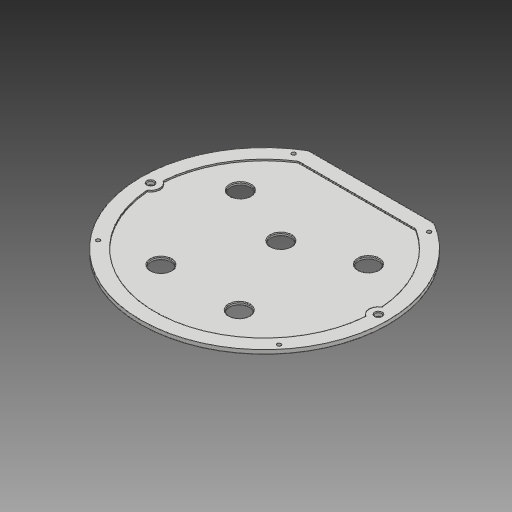
# Autodesk Inventor part: Gehäuse Unterplatte
Saved by Autodesk Inventor 2019.4 (Build 234330000, 330)
## iProperties
Part Number: Gehäuse Unterplatte
Material: Generisch
Document SubType Name: Modeling
Designer: rYan
Density: 1 g/cm^3
Appearance: Vorgabe
Mass: 48.9318 g
Surface Area: 477.374 cm^2
Volume: 48.9318 cm^3
Author: rYan
Autodesk Inventor part; units mm, degrees
ref_plane "YZ Plane" through (0, 0, 0) normal (1, 0, 0) x (0, 1, 0)
ref_plane "XZ Plane" through (0, 0, 0) normal (0, 1, 0) x (-1, 0, 0)
ref_plane "XY Plane" through (0, 0, 0) normal (0, 0, 1) x (1, 0, 0)
sketch "Skizze1" plane through (0, 0, 0) normal (0, 0, 1) x (1, 0, 0)
  arc A0 (-44.0908, 75) -> (44.0908, 75) centre (0, 0) ccw
  line L0 (-44.0908, 75) -> (44.0908, 75)
  dimension "d0" = 174
  dimension "d1" = 75
  constraints: 2 end point, 2 point on circle, 1 centre point, 1 coincident, 1 horizontal
  measures "d0" diameter of A0
  measures "d1" distance from line of point (0, 0) L0
extrude "Extrusion1" add sketch "Skizze1" along normal blind 2
sketch "Skizze2" plane through (0, 0, 2) normal (0, 0, 1) x (1, 0, 0)
  arc A0 (-44.0908, 75) -> (44.0908, 75) centre (0, 0) ccw projected
  line L0 (44.0908, 75) -> (-44.0908, 75) projected
  arc A1 (-41.2795, 65) -> (41.2795, 65) centre (0, 0) ccw
  line L1 (-41.2795, 65) -> (41.2795, 65)
  dimension "d4" = 10
  constraints: 2 end point, 2 point on circle, 1 centre point, 1 other
  measures "d4" radial gap between concentric circles of A0 A1
extrude "Extrusion2" add sketch "Skizze2" along normal blind 1
sketch "Skizze8" plane through (0, 0, 2) normal (0, 0, 1) x (1, 0, 0)
  line L0 (41.2795, 65) -> (-41.2795, 65) projected
  arc A0 (-41.2795, 65) -> (41.2795, 65) centre (0, 0) ccw projected
  circle A1 centre (0, 0) radius 80 construction
  circle A2 centre (-80, 0) radius 6.5
  circle A3 centre (80, 0) radius 6.5
  line L1 (-121.8, 0) -> (121.8, 0) projected
  dimension "d38" = 160
  dimension "d39" = 13
  dimension "d40" = 13
  constraints: 3 centre point, 2 point on circle, 2 point on line, 1 coincident
  measures "d38" diameter of A1
  measures "d39" diameter of A2
  measures "d40" diameter of A3
extrude "Extrusion4" add sketch "Skizze8" along normal blind 1 contours A3 L1 A0 | A0 L1 A3 | A2 L1 A0 | A0 L1 A2 | L1 A3 A0 | A0 A3 L1 | L1 A2 A0 | A0 A2 L1
sketch "Skizze3" plane through (0, 0, 3) normal (0, 0, 1) x (1, 0, 0)
  line L0 (0, 107.4) -> (0, -119.4) projected
  line L1 (-121.8, 0) -> (121.8, 0) projected
  point P0 (0, 0)
  point P1 (-80, 0)
  point P2 (80, 0)
  dimension "d7" = 160
  constraints: 2 point on line, 1 symmetric about line
  measures "d7" distance of point (80, 0) point (-80, 0)
hole "Bohrung1" at (-80, 0, 3) at (80, 0, 3) direction (0, 0, -1) diameter 4.4 end through all
sketch "Skizze4" plane through (0, 0, 3) normal (0, 0, 1) x (1, 0, 0)
  circle A0 centre (0, 0) radius 83 construction
  line L0 (0, 0) -> (-47.6068, 67.9896) construction
  line L1 (0, 0) -> (-63.5817, -53.3514) construction
  line L2 (0, 117) -> (0, -121) projected
  line L3 (-121.8, 0) -> (121.8, 0) projected
  point P0 (63.5817, -53.3514)
  point P1 (47.6068, 67.9896)
  dimension "d15" = 166
  dimension "d16" = 55
  dimension "d17" = 40
  constraints: 4 end point, 4 point on circle, 2 coincident, 2 symmetric about line, 1 centre point
  measures "d15" diameter of A0
  measures "d16" angle of L0 L3
  measures "d17" angle of L3 L1
hole "Bohrung2" at (-63.5817, -53.3514, 3) at (-47.6068, 67.9896, 3) at (63.5817, -53.3514, 3) at (47.6068, 67.9896, 3) direction (0, 0, -1) diameter 2.75 end through all
sketch "Skizze5" plane through (0, 0, 0) normal (0, 0, -1) x (-1, 0, 0)
  line L0 (0, -119.4) -> (0, 107.4) projected
  line L1 (-121.8, 0) -> (121.8, 0) projected
  point P0 (0, 0)
  point P1 (-45, 28)
  point P2 (-27.5, -45.25)
  point P3 (45, 28)
  point P4 (27.5, -45.25)
  point P5 (0, 11.5)
  dimension "d113" = 45
  dimension "d114" = 28
  dimension "d115" = 27.5
  dimension "d116" = 45.25
  dimension "d117" = 11.5
  constraints: 2 symmetric about line, 1 point on line
  measures "d113" distance from line of L0 point (-45, 28)
  measures "d114" distance from line of L1 point (-45, 28)
  measures "d115" distance from line of point (-27.5, -45.25) L0
  measures "d116" distance from line of point (-27.5, -45.25) L1
  measures "d117" distance from line of L1 point (0, 11.5)
hole "Bohrung3" at (45, 28, 0) at (27.5, -45.25, 0) at (0, 11.5, 0) at (-45, 28, 0) at (-27.5, -45.25, 0) direction (0, 0, 1) diameter 14 end through all
fillet "Rundung1" radius 2 4 edges at (-44.0908, 75, 1.5) (44.0908, 75, 1.5) (41.2795, 65, 2.5) (-41.2795, 65, 2.5)
sketch "Skizze17" plane through (0, 0, 0) normal (0, 0, -1) x (-1, 0, 0)
  line L0 (-43.5431, 75) -> (43.5431, 75) projected
  line L1 (28.5, 75) -> (-28.5, 75)
  line L2 (-28.5, 75) -> (-28.5, -28.5)
  line L3 (-28.5, -28.5) -> (28.5, -28.5)
  line L4 (28.5, -28.5) -> (28.5, 75)
  line L5 (0, -119.4) -> (0, 107.4) projected
  line L6 (-43.5431, 75) -> (43.5431, 75) projected
  line L7 (-30.5, 75) -> (30.5, 75)
  line L8 (30.5, 75) -> (30.5, -30.5)
  line L9 (30.5, -30.5) -> (-30.5, -30.5)
  line L10 (-30.5, -30.5) -> (-30.5, 75)
  point P0 (0, 0)
  point P1 (-5, 75)
  dimension "d107" = 28.5
  dimension "d108" = 57
  dimension "d109" = 2
  dimension "d110" = 2
  constraints: 16 end point, 4 parallel, 2 horizontal, 2 perpendicular, 2 point on line, 2 other
  measures "d107" distance from line of L3 point (0, 0)
  measures "d108" distance of L2.end L3.end
  measures "d109" distance between parallel lines of L10 L2
  measures "d110" distance between parallel lines of L3 L9
extrude "Extrusion10" cut sketch "Skizze17" against normal blind 1 contours L0 L2 L3 L5 L9 L10 | L5 L3 L4 L0 L8 L9
chamfer "Fase1" distance 0.3 angle 45 17 edges at (-27.5, -52.25, 0) (27.5, -52.25, 0) (-45, 21, 0) (45, 21, 0) (0, 4.5, 0) (-63.5817, -51.9764, 0) (63.5817, -51.9764, 0) (-47.6068, 69.3646, 0) (47.6068, 69.3646, 0) (-80, 2.2, 0) (80, 2.2, 0) (0, -87, 0) (44.0745, 74.9281, 0) (37.0215, 75, 0) (-44.0745, 74.9281, 0) (-37.0215, 75, 0) (0, 75, 0)
chamfer "Fase2" distance 0.5 angle 45 7 edges at (-27.5, -52.25, 2) (27.5, -52.25, 2) (-45, 21, 2) (0, 4.5, 2) (45, 21, 2) (-80, 2.2, 3) (80, 2.2, 3)
sketch "Skizze15" plane through (0, 0, 0) normal (0, 0, -1) x (-1, 0, 0)
  circle A0 centre (0, 0) radius 25
  circle A1 centre (54.772, 35) radius 20
  circle A2 centre (35, -54.772) radius 20
  circle A3 centre (-35, -54.772) radius 20
  circle A4 centre (-54.772, 35) radius 20
  line L0 (0, -119.4) -> (0, 107.4) projected
  line L1 (-121.8, 0) -> (121.8, 0) projected
  circle A5 centre (-54.772, 35) radius 20.5
  circle A6 centre (-35, -54.772) radius 20.5
  circle A7 centre (54.772, 35) radius 20.5
  circle A8 centre (35, -54.772) radius 20.5
  circle A9 centre (0, 0) radius 25.5
  dimension "d91" = 50
  dimension "d92" = 40
  dimension "d93" = 40
  dimension "d94" = 40
  dimension "d95" = 40
  dimension "d96" = 35
  dimension "d97" = 54.772
  dimension "d98" = 54.772
  dimension "d99" = 35
  dimension "d100" = 41
  dimension "d101" = 41
  dimension "d102" = 41
  dimension "d103" = 41
  dimension "d104" = 51
  constraints: 10 centre point, 6 coincident, 2 symmetric about line
  measures "d91" diameter of A0
  measures "d92" diameter of A1
  measures "d93" diameter of A2
  measures "d94" diameter of A3
  measures "d95" diameter of A4
  measures "d96" distance from line of A2.centre L0
  measures "d97" distance from line of L1 A2.centre
  measures "d98" distance from line of A1.centre L0
  measures "d99" distance from line of A1.centre L1
  measures "d100" diameter of A5
  measures "d101" diameter of A6
  measures "d102" diameter of A7
  measures "d103" diameter of A8
  measures "d104" diameter of A9
extrude "Extrusion9" cut sketch "Skizze15" against normal blind 0.2 contours A5 | A6 | A7 | A8
equation "\"d110\" = d109"
equation "\"d98\" = d97"
equation "\"d99\" = d96"
